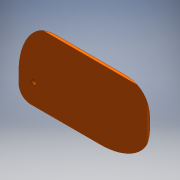
# Autodesk Inventor part: Loquet Lancement
Saved by Autodesk Inventor 2016 SP1 (Build 200210100, 210)
## iProperties
Created: 2017-04-27
Part Number: Loquet Lancement
Material: Plastique ABS
Document SubType Name: Modeling
Designer: dimercur
Density: 1.06 g/cm^3
Appearance: Lisse - Orange clair
Author: dimercur
Autodesk Inventor part; units mm, degrees
ref_plane "YZ Plane" through (0, 0, 0) normal (1, 0, 0) x (0, 1, 0)
ref_plane "XZ Plane" through (0, 0, 0) normal (0, 1, 0) x (-1, 0, 0)
ref_plane "XY Plane" through (0, 0, 0) normal (0, 0, 1) x (1, 0, 0)
sketch "Esquisse1" plane through (0, 0, 0) normal (0, 1, 0) x (-1, 0, 0)
  line L0 (-27.5, 15) -> (27.5, 15)
  line L1 (27.5, 15) -> (27.5, -15)
  line L2 (27.5, -15) -> (-27.5, -15)
  line L3 (-27.5, -15) -> (-27.5, 15)
  point P0 (0, 0)
  dimension "d0" = 55
  dimension "d1" = 30
  dimension "d2" = 15
  dimension "d3" = 27.5
  constraints: 8 end point, 2 parallel, 1 horizontal, 1 perpendicular
  measures "d0" distance of L0.start L0.end
  measures "d1" distance of L0.end L1.end
  measures "d2" vertical distance of point (0, 0) L0.end
  measures "d3" horizontal distance of point (0, 0) L0.end
extrude "Extrusion1" add sketch "Esquisse1" along normal blind 3
sketch "Esquisse2" plane through (0, 3, 0) normal (0, 1, 0) x (1, 0, 0)
  circle A0 centre (-21, 6) radius 6
  circle A1 centre (-21, 6) radius 2.75
  line L0 (-27.5, 15) -> (-27.5, -15) projected
  line L1 (27.5, 15) -> (-27.5, 15) projected
  point P0 (0, 0)
  dimension "d6" = 6.5
  dimension "d7" = 9
  dimension "d8" = 12
  dimension "d9" = 5.5
  constraints: 2 centre point, 1 coincident
  measures "d6" distance from line of L0 A0.centre
  measures "d7" distance from line of L1 A0.centre
  measures "d8" diameter of A0
  measures "d9" diameter of A1
extrude "Extrusion2" add sketch "Esquisse2" along normal blind 3
sketch "Esquisse3" plane through (-21, 3, -6) normal (0, 1, 0) x (1, 0, 0)
  circle A0 centre (0, 0) radius 2.75
  point P0 (21, -6)
  constraints: 1 centre point
extrude "Extrusion3" add sketch "Esquisse3" along normal blind 0.4
sketch "Esquisse4" plane through (-21, 3.4, -6) normal (0, 1, 0) x (1, 0, 0)
  circle A0 centre (0, 0) radius 1
  point P0 (21, -6)
  dimension "d14" = 2
  constraints: 1 centre point
  measures "d14" diameter of A0
extrude "Extrusion4" cut sketch "Esquisse4" against normal through all
chamfer "Chanfrein2" distance 1.9 angle 45 2 edges at (0, 3, 15) (27.5, 3, 0)
fillet "Congé5" radius 15 1 edges at (-27.5, 2.05, 14.05)
fillet "Congé6" radius 15 2 edges at (26.55, 2.05, 14.05) (26.55, 2.05, -15)
fillet "Congé7" radius 5 1 edges at (-27.5, 1.5, -15)
fillet "Congé8" radius 1 1 edges at (-27, 3, -6)
equation "\"d2\" = 0.5 * d1"
equation "\"d3\" = 0.5 * d0"
